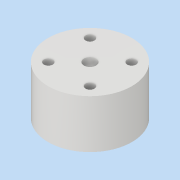
# Autodesk Inventor part: 1PieceAttachment
Saved by Autodesk Inventor 2017 (Build 210142000, 142)
## iProperties
Created: 2016-11-03
Part Number: 1PieceAttachment
Material: ABS Plastic
Document SubType Name: Modeling
Designer: techn
Density: 1.06 g/cm^3
Appearance: Smooth - White
Author: techn
Autodesk Inventor part; units mm, degrees
ref_plane "YZ Plane" through (0, 0, 0) normal (1, 0, 0) x (0, 1, 0)
ref_plane "XZ Plane" through (0, 0, 0) normal (0, 1, 0) x (-1, 0, 0)
ref_plane "XY Plane" through (0, 0, 0) normal (0, 0, 1) x (1, 0, 0)
sketch "Sketch1" plane through (0, 0, 0) normal (0, 1, 0) x (-1, 0, 0)
  circle A0 centre (0, 0) radius 12.065
  line L0 (0, 0) -> (6.0168, -6.0168)
  line L1 (0, 0) -> (8.509, 0) construction
  circle A1 centre (6.0168, -6.0168) radius 1.27
  circle A2 centre (6.0168, 6.0168) radius 1.27
  circle A3 centre (-6.0168, 6.0168) radius 1.27
  circle A4 centre (-6.0168, -6.0168) radius 1.27
  dimension "d0" = 24.13
  dimension "d1" = 45
  dimension "d2" = 8.509
  dimension "d3" = 2.54
  dimension "d6" = 360
  constraints: 5 centre point, 4 end point, 2 coincident, 1 equal length, 1 horizontal, 9 other
  measures "d0" diameter of A0
  measures "d1" angle of L0 L1
  measures "d2" distance of L0.start L0.end
  measures "d3" diameter of A1
extrude "Extrusion1" add sketch "Sketch1" along normal blind 13.97
sketch "Sketch6" plane through (0, 13.97, 0) normal (0, 1, 0) x (1, 0, 0)
  circle A0 centre (0, 0) radius 1.75
  dimension "d32" = 3.5
  constraints: 1 centre point, 1 coincident
  measures "d32" diameter of A0
extrude "Extrusion3" cut sketch "Sketch6" against normal through all
sketch "Sketch3" plane through (0, 13.97, 0) normal (0, 1, 0) x (1, 0, 0)
  circle A0 centre (0, 0) radius 1.75
  dimension "d14" = 3.5
  constraints: 1 centre point, 1 coincident
  measures "d14" diameter of A0
sketch "Sketch7" plane through (0, 0, 0) normal (0, 0, 1) x (1, 0, 0)
  arc A0 (0, 13.97) -> (7.9375, 6.0325) centre (7.9375, 13.97) ccw
  line L0 (7.9375, 6.0325) -> (8.1915, 6.0325)
  point P0 (0, 0)
  dimension "d27" = 7.9375
  dimension "d28" = 7.9375
  dimension "d31" = 0.254
  constraints: 2 end point, 2 point on circle, 1 centre point, 1 horizontal, 1 tangent
  measures "d27" horizontal distance of L0.start A0.start
  measures "d28" horizontal distance of A0.start L0.start
  measures "d31" distance of L0.start L0.end
sweep "Sweep2" cut profiles "Sketch3" path "Sketch7"
body "Solid1"
